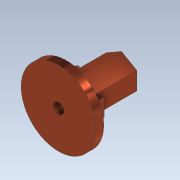
# Autodesk Inventor part: Coupling_0515
Saved by Autodesk Inventor 2022 (Build 260153000, 153)
## iProperties
Created: 2023-05-15
Part Number: Coupling_0515
Material: 一般
Document SubType Name: Modeling
Designer: Johnny Jou
Density: 1 g/cm^3
Appearance: 預設
Author: Johnny Jou
Autodesk Inventor part; units mm, degrees
ref_plane "YZ Plane" through (0, 0, 0) normal (1, 0, 0) x (0, 1, 0)
ref_plane "XZ Plane" through (0, 0, 0) normal (0, 1, 0) x (-1, 0, 0)
ref_plane "XY Plane" through (0, 0, 0) normal (0, 0, 1) x (1, 0, 0)
sketch "草圖1" plane through (0, 0, 0) normal (0, 0, 1) x (1, 0, 0)
  line L0 (-5.85, 3.3775) -> (0, 6.755)
  line L1 (0, 6.755) -> (5.85, 3.3775)
  line L2 (5.85, 3.3775) -> (5.85, -3.3775)
  line L3 (5.85, -3.3775) -> (0, -6.755)
  line L4 (0, -6.755) -> (-5.85, -3.3775)
  line L5 (-5.85, -3.3775) -> (-5.85, 3.3775)
  point P0 (0, 0)
  point P1 (0, 0)
  dimension "d0" = 11.7
  constraints: 12 end point, 1 coincident, 1 vertical, 13 other
  measures "d0" distance between parallel lines of L2 L5
extrude "擠出1" add sketch "草圖1" along normal blind 24
sketch "草圖2" plane through (0, 0, 24) normal (0, 0, 1) x (1, 0, 0)
  circle A0 centre (0, 0) radius 14.25
  dimension "d3" = 28.5
  constraints: 1 centre point, 1 coincident
  measures "d3" diameter of A0
extrude "擠出2" add sketch "草圖2" against normal blind 3
sketch "草圖3" plane through (0, 0, 21) normal (0, 0, -1) x (-1, 0, 0)
  line L0 (5.85, -3.3775) -> (0, -6.755) projected
  line L1 (5.85, 3.3775) -> (5.85, -3.3775) projected
  line L2 (0, 6.755) -> (5.85, 3.3775) projected
  line L3 (-5.85, 3.3775) -> (0, 6.755) projected
  line L4 (-5.85, -3.3775) -> (-5.85, 3.3775) projected
  line L5 (0, -6.755) -> (-5.85, -3.3775) projected
  line L6 (-5.85, 3.3775) -> (0, 6.755) projected
  line L7 (0, 6.755) -> (5.85, 3.3775) projected
  line L8 (0, 6.755) -> (5.85, 3.3775)
  line L9 (5.85, 3.3775) -> (7.1, 5.5426)
  line L10 (7.1, 5.5426) -> (1.25, 8.9201)
  line L11 (1.25, 8.9201) -> (0, 6.755)
  line L12 (-5.85, -3.3775) -> (-5.85, 3.3775)
  line L13 (-5.85, 3.3775) -> (-8.35, 3.3775)
  line L14 (-8.35, 3.3775) -> (-8.35, -3.3775)
  line L15 (-8.35, -3.3775) -> (-5.85, -3.3775)
  line L16 (5.85, -3.3775) -> (0, -6.755)
  line L17 (0, -6.755) -> (1.25, -8.9201)
  line L18 (1.25, -8.9201) -> (7.1, -5.5426)
  line L19 (7.1, -5.5426) -> (5.85, -3.3775)
  point P0 (0, 0)
  point P1 (0, -6.755)
  dimension "d6" = 2.5
  dimension "d9" = 360
  constraints: 24 end point, 3 equal length, 1 perpendicular, 25 other
  measures "d6" distance of L1.start L9.end
extrude "擠出3" add sketch "草圖3" along normal blind 6 contours L19 L18 L17 L0 | L2 L11 L10 L9 | L15 L14 L13 L4
sketch "草圖4" plane through (0, 0, 0) normal (0, 0, -1) x (-1, 0, 0)
  circle A0 centre (0, 0) radius 2
  dimension "d13" = 4
  constraints: 1 centre point, 1 coincident
  measures "d13" diameter of A0
extrude "擠出4" cut sketch "草圖4" against normal up to surface (24 mm away)
sketch "草圖5" plane through (0, 0, 0) normal (0, 0, -1) x (-1, 0, 0)
  circle A0 centre (0, 0) radius 2 projected
  circle A1 centre (0, 0) radius 2.05
  dimension "d16" = 4.1
  constraints: 1 centre point, 1 coincident
  measures "d16" diameter of A1
extrude "擠出5" cut sketch "草圖5" against normal blind 8 contours A0 | A1
sketch "草圖6" plane through (5.85, 3.3775, 15) normal (0.5, 0.8660254, 0) x (0.8660254, -0.5, 0)
  line L0 (10.8725, -6) -> (-17.6275, -6) projected
  circle A0 centre (-3.3775, -4) radius 1.5
  line L1 (-3.3775, 19.8) -> (-3.3775, -13.8) projected
  point P0 (-3.3775, 15)
  dimension "d19" = 3
  dimension "d22" = 2
  constraints: 1 centre point, 1 point on line
  measures "d19" diameter of A0
  measures "d22" distance from line of L0 A0.centre
extrude "擠出6" cut sketch "草圖6" against normal blind 6
sketch "草圖7" plane through (5.85, 3.3775, 15) normal (0.5, 0.8660254, 0) x (0.8660254, -0.5, 0)
  circle A0 centre (-3.3775, -4) radius 1.5 projected
  circle A1 centre (-3.3775, -4) radius 1.55
  point P0 (-3.3775, 15)
  dimension "d23" = 3.1
  constraints: 1 centre point, 1 coincident
  measures "d23" diameter of A1
extrude "擠出7" cut sketch "草圖7" against normal blind 6 contours A0 | A1
